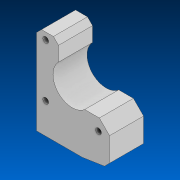
# Autodesk Inventor part: y-stepper-mount
Saved by Autodesk Inventor 2021 (Build 250183000, 183)
## iProperties
Created: 2021-03-10
Part Number: y-stepper-mount
Material: Generic
Document SubType Name: Modeling
Designer: Alex
Density: 1 g/cm^3
Appearance: Default
Author: Alex
Autodesk Inventor part; units mm, degrees
ref_plane "YZ Plane" through (0, 0, 0) normal (1, 0, 0) x (0, 1, 0)
ref_plane "XZ Plane" through (0, 0, 0) normal (0, 1, 0) x (-1, 0, 0)
ref_plane "XY Plane" through (0, 0, 0) normal (0, 0, 1) x (1, 0, 0)
sketch "Sketch1" plane through (0, 0, 0) normal (0, 0, 1) x (1, 0, 0)
  line L0 (0, 0) -> (3, 3)
  line L1 (3, 3) -> (10, 3)
  line L2 (10, 3) -> (13, 0)
  line L3 (13, 0) -> (13, -8.5904)
  circle A0 centre (21, -16.5) radius 11.25
  line L4 (28.3697, -25) -> (37, -25)
  line L5 (37, -25) -> (43, -31)
  line L6 (43, -31) -> (43, -45)
  line L7 (43, -45) -> (40, -48)
  line L8 (40, -48) -> (27, -50)
  line L9 (27, -50) -> (0, -50)
  line L10 (0, -50) -> (0, 0)
  circle A1 centre (5.5, -1) radius 1.7
  circle A2 centre (5.5, -32) radius 1.7
  circle A3 centre (36.5, -32) radius 1.7
  line L11 (5.5, -32) -> (5.5, -1) construction
  line L12 (5.5, -32) -> (36.5, -32) construction
  dimension "d0" = 16.5
  dimension "d1" = 21
  dimension "d2" = 50
  dimension "d3" = 22.5
  dimension "d4" = 8
  dimension "d5" = 45
  dimension "d6" = 3
  dimension "d7" = 8.5
  dimension "d8" = 6
  dimension "d9" = 3
  dimension "d10" = 13
  dimension "d11" = 22
  dimension "d12" = 2
  dimension "d14" = 3.4
  dimension "d15" = 15.5
  dimension "d16" = 31
  dimension "d17" = 31
  dimension "d18" = 15.5
  constraints: 26 end point, 7 perpendicular, 4 centre point, 3 horizontal, 2 equal radius, 2 point on circle, 1 parallel, 1 vertical
  measures "d0" vertical distance of A0.centre L0.start
  measures "d1" horizontal distance of A0.centre L0.start
  measures "d2" distance of L9.end L0.start
  measures "d3" diameter of A0
  measures "d4" distance from line of A0.centre L3
  measures "d5" angle of L1 L0
  measures "d6" distance from line of L0.start L1
  measures "d7" distance from line of L4 A0.centre
  measures "d8" horizontal distance of L4.end L5.end
  measures "d9" horizontal distance of L6.end L7.end
  measures "d10" horizontal distance of L7.end L8.end
  measures "d11" distance from line of L6 A0.centre
  measures "d12" vertical distance of L7.end L8.end
  measures "d14" diameter of A1
  measures "d15" horizontal distance of L11.start A0.centre
  measures "d16" distance of L11.start L11.end
  measures "d17" distance of L12.end L11.start
  measures "d18" horizontal distance of L11.start A0.centre
extrude "Extrusion1" add sketch "Sketch1" along normal mid plane 20 contours L0 L1 L2 L3 A0 L4 L5 L6 L7 L8 L9 L10
equation "\"d17\" = d16"
body "Solid1"
